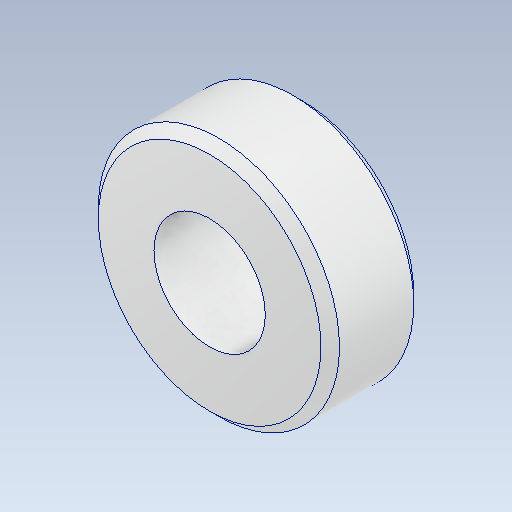
# Autodesk Inventor part: 686_bearing
Saved by Autodesk Inventor 2020 (Build 240168000, 168)
## iProperties
Created: 2021-04-05
Part Number: 686_bearing
Material: Aluminum 6061
Document SubType Name: Modeling
Designer: patry
Density: 2.7 g/cm^3
Appearance: Aluminum - Flat
Mass: 1.38332 g
Surface Area: 4.82793 cm^2
Volume: 0.512341 cm^3
Author: patry
Autodesk Inventor part; units mm, degrees
ref_plane "YZ Plane" through (0, 0, 0) normal (1, 0, 0) x (0, 1, 0)
ref_plane "XZ Plane" through (0, 0, 0) normal (0, 1, 0) x (-1, 0, 0)
ref_plane "XY Plane" through (0, 0, 0) normal (0, 0, 1) x (1, 0, 0)
sketch "Szkic1" plane through (0, 0, 0) normal (0, 0, 1) x (1, 0, 0)
  circle A0 centre (0, 0) radius 3
  circle A1 centre (0, 0) radius 6.5
  dimension "d0" = 6
  dimension "d1" = 13
  constraints: 2 centre point, 2 coincident
  measures "d0" diameter of A0
  measures "d1" diameter of A1
extrude "Wyciągnięcie proste1" add sketch "Szkic1" along normal blind 5
chamfer "Faza1" distance 0.5 angle 45 1 edges at (-6.5, 0, 5)
chamfer "Faza2" distance 0.5 angle 45 1 edges at (-6.5, 0, 0)
